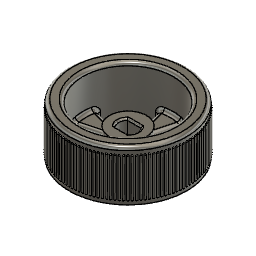
Arduino wheel (Autodesk Fusion 360 design; units mm, degrees)
Autodesk Fusion 360 part; units mm, degrees
note: some values were not read from the file. Chosen so that the rebuilt part matches the saved one: which face or edge a step refers to. Set by a fixed rule: which sketch regions a step uses.
sketch "Sketch1" plane through (0, 0, 0) normal (0, 1, 0) x (1, 0, 0)
  circle A0 centre (0, 0) radius 17.5
  circle A1 centre (0, 0) radius 13.5
  circle A2 centre (0, 0) radius 5.5
  line L0 (-2.07, 1.8855) -> (2.07, 1.8855)
  line L1 (-2.0432, -1.9145) -> (2.0432, -1.9145)
  line L2 (-0.0541, -0.0145) -> (0.0541, -0.0145)
  arc A3 (-2.07, 1.8855) -> (-2.0432, -1.9145) centre (0, 0) ccw
  arc A4 (2.0432, -1.9145) -> (2.07, 1.8855) centre (0, 0) ccw
  line L3 (-0.0039, -0.0145) -> (0, 0)
  line L4 (3.4941, -13.04) -> (1.4235, -5.3126)
  line L5 (0.0039, -0.0145) -> (0, 0)
  line L6 (13.0741, -3.5032) -> (5.3126, -1.4235)
  line L7 (0.0541, -0.0145) -> (0, 0)
  line L8 (3.4941, 13.04) -> (1.4235, 5.3126)
  line L9 (-3.4941, 13.04) -> (-1.4235, 5.3126)
  line L10 (-13.057, 3.4986) -> (-5.3126, 1.4235)
  line L11 (-13.0759, -3.5037) -> (-5.3126, -1.4235)
  line L12 (-0.0541, -0.0145) -> (0, 0)
  line L13 (-1.4235, -5.3126) -> (-3.4941, -13.04)
  line L14 (5.3126, 1.4235) -> (13.0741, 3.3642)
  dimension "d1" = 35
  dimension "d2" = 27
  dimension "d3" = 11
  dimension "d4" = 5.6
  dimension "d6" = 1.9
  dimension "d7" = 1.9
  constraint coincident A0.centre A1.centre
  constraint concentric A0 A1
  constraint concentric A0 A2
  constraint concentric A1 A3
  constraint horizontal L0
  constraint coincident L1.end A3
  constraint parallel L0 L1
  constraint parallel L1 L2
  constraint concentric A3 A4
  constraint coincident A1 L8.start
  constraint coincident A1 L9.start
  constraint coincident A1 L4.start
  constraint coincident A2 L4.end
  constraint collinear L4 L5
  constraint coincident A2 L6.end
  constraint collinear L6 L7
  constraint coincident A2 L8.end
  constraint coincident A2 L9.end
  constraint coincident A2 L10.end
  constraint coincident A2 L11.end
  constraint collinear L11 L12
  constraint coincident L2 L3.start
  constraint coincident L2 L5.start
  constraint coincident A2 L13.start
  constraint coincident A1 L13.end
  constraint coincident A2 L14.start
  constraint coincident A1 L14.end
  measures "d1" diameter of A0
  measures "d2" diameter of A1
  measures "d3" diameter of A2
  measures "d4" diameter of A3
  measures "d6" distance of L0 L2
  measures "d7" distance of L1 L2
extrude "Extrude1" add sketch "Sketch1" along normal blind 4 contours A1 A2 L6 L14 | A1 A2 L8 L9 | A1 A2 L4 L13 | A1 A2 L10 L11 makes body 1 at (-2.2266, 0, -10.579) makes body 2 at (10.6414, 0, -1.9147) makes body 3 at (-10.579, 0, -2.2266) makes body 4 at (1.9914, 0, 10.6258)
extrude "Extrude2" add sketch "Sketch1" along normal blind 15 contours A0 bodies 1 2 3 4
extrude "Extrude3" add sketch "Sketch1" along normal blind 8 contours A2 bodies 1
fillet "Fillet1" radius 1 10 edges at (-9.1763, 4, -2.4588) (-9.1763, 4, 2.4588) (-2.4588, 4, -9.1763) (2.4588, 4, -9.1763) (9.1934, 4, -2.3938) (9.1763, 4, 2.4588) (2.4588, 4, 9.1763) (-2.4588, 4, 9.1763) (-12.5864, 15, -4.8818) (-16.3157, 15, 6.3283) on bodies 1
fillet "Fillet2" radius 1 10 edges at (3.4941, 1.5, -13.04) (3.21, 3.7074, -13.1128) (0, 4, -13.5) (-3.21, 3.7074, -13.1128) (-3.4941, 1.5, -13.04) (-13.04, 1.5, 3.4941) (-13.1128, 3.7074, 3.21) (-13.5, 4, 0) (-13.1128, 3.7074, -3.21) (-13.04, 1.5, -3.4941) on bodies 1
fillet "Fillet3" radius 1 10 edges at (13.0741, 1.5, -3.3642) (13.1441, 3.7073, -3.0795) (13.4998, 4, 0.067) (13.1128, 3.7074, 3.21) (13.04, 1.5, 3.4941) (3.4941, 1.5, 13.04) (3.21, 3.7074, 13.1128) (0, 4, 13.5) (-3.21, 3.7074, 13.1128) (-3.4941, 1.5, 13.04) on bodies 1
fillet "Fillet4" radius 0.5 4 edges at (0, 8, -1.8855) (-2.7999, 8, 0.0198) (0, 8, 1.9145) (2.7999, 8, 0.0198) on bodies 1
sketch "Sketch2" plane through (0, 0, 0) normal (1, 0, 0) x (0, 0, -1)
ref_plane "WorkPlane1" through (0, 1, 0) normal (0, 1, 0) x (1, 0, 0)
sketch "Sketch3" plane through (0, 1, 0) normal (0, 1, 0) x (1, 0, 0)
  circle A0 centre (17.5, 0) radius 0.25
  line L0 (17.5009, 0.25) -> (17.5009, -0.25)
  dimension "d27" = 0.5
  constraint coincident A0 L0.start
  constraint coincident A0 L0.end
  constraint vertical L0
  measures "d27" diameter of A0
extrude "Extrude4" add sketch "Sketch3" along normal blind 12 separate body contours A0 L0 picked at (17.5949, 0.0109) makes body 5
fillet "Fillet5" radius 0.25 2 edges at (17.6771, 13, 0.1765) (17.6771, 13, -0.1765) on bodies 5
fillet "Fillet6" radius 0.25 1 edges at (17.75, 1, 0) on bodies 5
pattern_circular "C-Pattern1" count 120 over 360 about axis through (0, 0, 0) along (0, 1, 0) of bodies 5 makes body 6 at (17.4887, 8.9171, -1.1656) makes body 7 at (17.4409, 8.9171, -2.0765) makes body 8 at (17.4471, 8.9171, -2.5477) makes body 9 at (17.2243, 8.9171, -3.8646) makes body 10 at (17.0476, 5.0829, -4.3249) makes body 11 at (16.7917, 8.9171, -5.6091) makes body 12 at (16.2606, 8.9171, -6.5093) makes body 13 at (16.0444, 8.9171, -7.3612) makes body 14 at (15.6001, 5.0829, -8.1947) makes body 15 at (15.4051, 5.0829, -8.7627) makes body 16 at (14.6333, 5.0829, -9.7774) makes body 17 at (14.4067, 8.9171, -10.263) makes body 18 at (13.7765, 8.9171, -10.836) makes body 19 at (13.1058, 5.0829, -11.9386) makes body 20 at (12.463, 5.0829, -12.6081) makes body 21 at (11.9386, 8.9171, -13.1058) makes body 22 at (10.836, 5.0829, -13.7765) makes body 23 at (10.263, 5.0829, -14.4067) makes body 24 at (9.7774, 8.9171, -14.6333) makes body 25 at (8.7254, 8.9171, -15.4042) makes body 26 at (8.194, 8.9171, -15.6125) makes body 27 at (6.9977, 8.9171, -16.2062) makes body 28 at (6.5093, 5.0829, -16.2606) makes body 29 at (5.6091, 5.0829, -16.7917) makes body 30 at (4.3249, 8.9171, -17.0476) makes body 31 at (3.874, 8.9171, -17.2013) makes body 32 at (2.5477, 8.9171, -17.4471) makes body 33 at (2.0792, 8.9171, -17.4037) makes body 34 at (1.1659, 5.0829, -17.4762) makes body 35 at (-0.199, 8.9171, -17.6514) makes body 36 at (-1.1656, 8.9171, -17.4887) makes body 37 at (-2.0765, 8.9171, -17.4409) makes body 38 at (-2.4931, 5.0829, -17.3367) makes body 39 at (-3.8646, 8.9171, -17.2243) makes body 40 at (-4.3249, 5.0829, -17.0476) makes body 41 at (-5.6091, 8.9171, -16.7917) makes body 42 at (-6.5093, 8.9171, -16.2606) makes body 43 at (-6.9977, 5.0829, -16.2062) makes body 44 at (-8.1947, 5.0829, -15.6001) makes body 45 at (-8.7751, 5.0829, -15.4042) makes body 46 at (-9.7749, 5.0829, -14.6211) makes body 47 at (-10.496, 8.9171, -14.0218) makes body 48 at (-10.836, 8.9171, -13.7765) makes body 49 at (-11.9386, 5.0829, -13.1058) makes body 50 at (-12.6081, 5.0829, -12.463) makes body 51 at (-13.1058, 8.9171, -11.9386) makes body 52 at (-13.7765, 5.0829, -10.836) makes body 53 at (-14.4067, 5.0829, -10.263) makes body 54 at (-14.5519, 5.0829, -9.7478) makes body 55 at (-15.4042, 8.9171, -8.7254) makes body 56 at (-15.7486, 5.0829, -7.7495) makes body 57 at (-16.0799, 5.0829, -7.35) makes body 58 at (-16.334, 5.0829, -6.5214) makes body 59 at (-16.8015, 5.0829, -5.6015) makes body 60 at (-17.0476, 8.9171, -4.3249) makes body 61 at (-17.1283, 8.9171, -3.8882) makes body 62 at (-17.4374, 5.0829, -2.5398) makes body 63 at (-17.4409, 8.9171, -2.0765) makes body 64 at (-17.4762, 5.0829, -1.1659) makes body 65 at (-17.6514, 8.9171, 0.199) makes body 66 at (-17.4762, 8.9171, 1.1659) makes body 67 at (-17.4409, 8.9171, 2.0765) makes body 68 at (-17.4471, 8.9171, 2.5477) makes body 69 at (-17.1894, 5.0829, 3.8779) makes body 70 at (-17.0476, 5.0829, 4.3249) makes body 71 at (-16.7917, 8.9171, 5.6091) makes body 72 at (-16.334, 8.9171, 6.5214) makes body 73 at (-16.0444, 8.9171, 7.3612) makes body 74 at (-15.7581, 8.9171, 7.7575) makes body 75 at (-15.4051, 5.0829, 8.7627) makes body 76 at (-14.6333, 5.0829, 9.7774) makes body 77 at (-14.0218, 8.9171, 10.496) makes body 78 at (-13.7765, 8.9171, 10.836) makes body 79 at (-13.1058, 5.0829, 11.9386) makes body 80 at (-12.4513, 5.0829, 12.6122) makes body 81 at (-11.9433, 8.9171, 13.0943) makes body 82 at (-10.836, 5.0829, 13.7765) makes body 83 at (-10.263, 5.0829, 14.4067) makes body 84 at (-9.7774, 8.9171, 14.6333) makes body 85 at (-8.7254, 8.9171, 15.4042) makes body 86 at (-8.1883, 8.9171, 15.6493) makes body 87 at (-7.3581, 8.9171, 16.0564) makes body 88 at (-6.5114, 5.0829, 16.4076) makes body 89 at (-5.6091, 5.0829, 16.7917) makes body 90 at (-4.3249, 8.9171, 17.0476) makes body 91 at (-3.874, 8.9171, 17.2013) makes body 92 at (-2.5398, 5.0829, 17.4374) makes body 93 at (-2.0792, 8.9171, 17.4037) makes body 94 at (-1.1656, 8.9171, 17.4887) makes body 95 at (-0.199, 5.0829, 17.6514) makes body 96 at (1.1656, 8.9171, 17.4887) makes body 97 at (1.5824, 5.0829, 17.4434) makes body 98 at (2.4931, 5.0829, 17.3367) makes body 99 at (3.8646, 8.9171, 17.2243) makes body 100 at (4.3323, 8.9171, 17.0576) makes body 101 at (5.6091, 8.9171, 16.7917) makes body 102 at (6.5093, 8.9171, 16.2606) makes body 103 at (6.9977, 5.0829, 16.2062) makes body 104 at (8.1947, 5.0829, 15.6001) makes body 105 at (8.7627, 5.0829, 15.4051) makes body 106 at (9.7793, 5.0829, 14.7077) makes body 107 at (10.496, 8.9171, 14.0218) makes body 108 at (10.836, 8.9171, 13.7765) makes body 109 at (11.9589, 8.9171, 12.9844) makes body 110 at (12.6081, 5.0829, 12.463) makes body 111 at (13.1058, 8.9171, 11.9386) makes body 112 at (13.7765, 5.0829, 10.836) makes body 113 at (14.4067, 5.0829, 10.263) makes body 114 at (14.6333, 8.9171, 9.7774) makes body 115 at (15.4042, 8.9171, 8.7254) makes body 116 at (15.6125, 8.9171, 8.194) makes body 117 at (16.0564, 8.9171, 7.3581) makes body 118 at (16.3464, 8.9171, 6.5213) makes body 119 at (16.8015, 5.0829, 5.6015) makes body 120 at (17.0476, 8.9171, 4.3249) makes body 121 at (17.2013, 8.9171, 3.874) makes body 122 at (17.4374, 5.0829, 2.5398) makes body 123 at (17.4037, 8.9171, 2.0792) makes body 124 at (17.4762, 5.0829, 1.1659)
equation "d6 = ( 3.8 / 2 ) * 1 mm"
